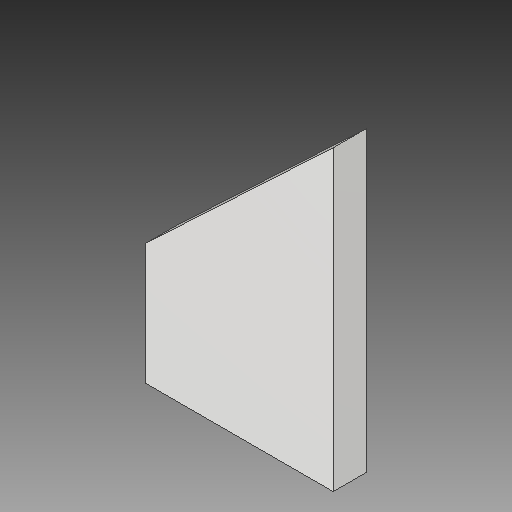
# Autodesk Inventor part: aletas
Saved by Autodesk Inventor 2018 (Build 220112000, 112)
## iProperties
Created: 2018-04-02
Part Number: aletas
Material: ABS plástico
Document SubType Name: Modeling
Designer: Ernandes
Density: 1.06 g/cm^3
Appearance: Liso - Branco
Author: Ernandes
Autodesk Inventor part; units mm, degrees
ref_plane "YZ Plane" through (0, 0, 0) normal (1, 0, 0) x (0, 1, 0)
ref_plane "XZ Plane" through (0, 0, 0) normal (0, 1, 0) x (-1, 0, 0)
ref_plane "XY Plane" through (0, 0, 0) normal (0, 0, 1) x (1, 0, 0)
sketch "Esboço1" plane through (0, 0, 0) normal (0, 0, 1) x (1, 0, 0)
  line L0 (0, 0) -> (17, 0)
  line L1 (0, 0) -> (0, 11)
  line L2 (17, 0) -> (17, 11)
  line L3 (17, 11) -> (17, 27)
  line L4 (17, 27) -> (0, 11)
  dimension "d0" = 17
  dimension "d1" = 11
  dimension "d2" = 16
  constraints: 10 end point, 2 vertical, 1 horizontal, 1 point on line
  measures "d0" distance of L0.start L0.end
  measures "d1" distance of L0.start L1.end
  measures "d2" distance of L2.end L3.end
extrude "Extrusão1" add sketch "Esboço1" along normal blind 3
